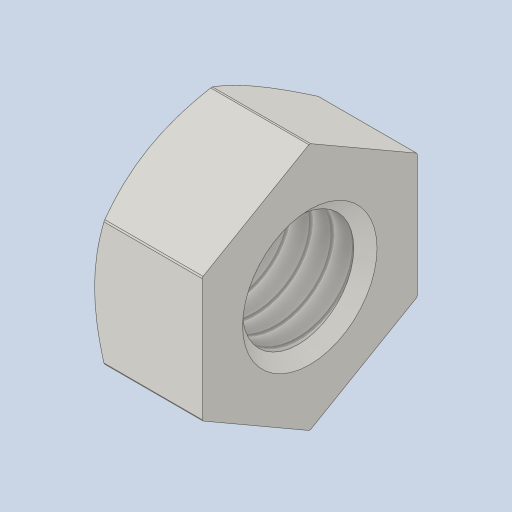
# Autodesk Inventor part: SLBNR5
Saved by Autodesk Inventor 2023 (Build 270158000, 158)
## iProperties
Category: PARTsolutions
Company: MISUMI
Created: 2024-11-13
Part Number: SLBNR5
Material: 鋼
Catalog Web Link: www.cadenas.de
Description: LBNR, LBNL, SLBNR, SLBNL, KNTR, KNTL, SKNTR-Nuts
Vendor: MISUMI
Document SubType Name: Modeling
Designer: psAdmin
Manufacturer: MISUMI
Mass: 1.29398 g
Surface Area: 2.37881 cm^2
Volume: 0.164839 cm^3
Density: 7.85 g/cm^3
Appearance: 鋼
PSOL_IDENT_0: {$CADENAS_DATA/23d-libs/misumi/metric/27_screws_nuts/slbnl.prj},199 {VTYP=3D},{NB=SLBNR5},{LINA=SLBN
PSOL_IDENT_1: R5},{NN=LBNR, LBNL, SLBNR, SLBNL, KNTR, KNTL, SKNTR},{DATE=30.06.2021 13:09:40},{GEOMDATE=05.11.2010
PSOL_IDENT_2: 00:00:00},{VERSION=},{LINEID=40},{WBVAR=TRS,MAT,CS},{WBNUMERIC=}  {NB=SLBNR5},{LINA=SLBNR5},{KT=DUM
PSOL_IDENT_3: MY},{PN=SLBNR5},{TS=LBN},{TRS=R},{MAT=S},{ST=-},{CS=1},{M1=5},{M=5.0},{P=0.80},{B=8.0},{EE=9.2},{T=4
PSOL_IDENT_4: .0},{T1=0.0},{TFX=4.0},{T1FX=3.2},{CALG='1','JIS Class 1','2','JIS Class 3'},{TRSALG= 'R', 'Right-Ha
PSOL_IDENT_5: nd Thread', 'L', 'Left-Hand Thread' },{MATALG= '', 'SWCH Carbon Steel', 'S', '304 Stainless Steel' }
NB: SLBNR5
NN: LBNR, LBNL, SLBNR, SLBNL, KNTR, KNTL, SKNTR
NT: Nuts
NBSYN: $PN.
LINA: SLBNR5
CATALOG: Misumi
PN: SLBNR5
TRS: Right-Hand Thread
MAT: 304 Stainless Steel Equivalent
ST: -
CS: JIS Class 1
M1: 5
P: 0.8
B: 8
EE: 9.2
T: 4
T1: 0
SUPPLIER: MISUMI
ARTICLENO: SLBNR5
BOMINFO: SLBNR5
CREATOR: CADENAS GmbH
Title: SLBNR5
Author: Cadenas PARTsolutions
Comments: Nuts
Autodesk Inventor part; units mm, degrees
sketch "Sketch_1" plane through (0, 0, 0) normal (0, 0, 1) x (1, 0, 0)
  line L0 (2, 0) -> (-2, 0)
  line L1 (-2, 0) -> (-2, 4)
  line L2 (-2, 4) -> (-1.6536, 4.6)
  line L3 (-1.6536, 4.6) -> (2, 4.6)
  line L4 (2, 4.6) -> (2, 0)
  line L5 (2, 0) -> (-2, 0)
  constraints: 12 end point
revolve "Revolution1" add sketch "Sketch_1" angle 360 about axis through (2, 0, 0) along (1, 0, 0)
sketch "Sketch_2" plane through (0, 0, 0) normal (0, 0, 1) x (1, 0, 0)
  line L0 (2, 0) -> (-2, 0)
  line L1 (-2, 0) -> (-2, 2.5)
  line L2 (-2, 2.5) -> (-1.567, 2.067)
  line L3 (-1.567, 2.067) -> (1.567, 2.067)
  line L4 (1.567, 2.067) -> (2, 2.5)
  line L5 (2, 2.5) -> (2, 0)
  line L6 (2, 0) -> (-2, 0)
  constraints: 14 end point
revolve "Revolution2" cut sketch "Sketch_2" angle 360 about axis through (2, 0, 0) along (1, 0, 0)
thread "Thread1" size "M5x0.8" class "6H" standard "ISO Metric profile" full length
sketch "Sketch_3" plane through (0, 0, 0) normal (1, 0, 0) x (0, 1, 0)
  line L0 (-8, 8) -> (-8, -8)
  line L1 (-8, -8) -> (8, -8)
  line L2 (8, -8) -> (8, 8)
  line L3 (8, 8) -> (-8, 8)
  line L4 (-2.3094, 4) -> (-4.6188, 0)
  line L5 (-4.6188, 0) -> (-2.3094, -4)
  line L6 (-2.3094, -4) -> (2.3094, -4)
  line L7 (2.3094, -4) -> (4.6188, 0)
  line L8 (4.6188, 0) -> (2.3094, 4)
  line L9 (2.3094, 4) -> (-2.3094, 4)
  constraints: 20 end point
extrude "Extrusion1" cut sketch "Sketch_3" along normal mid plane 4
ref_plane "cp_XY" through (2, 0, 0) normal (1, 0, 0) x (0, 0, -1)
ref_plane "cp_YZ" through (2, 0, 0) normal (0, 0, -1) x (0, 1, 0)
ref_plane "cp_ZX" through (2, 0, 0) normal (0, 1, 0) x (1, 0, 0)
ref_plane "nut_to_screw_XY" through (0, 0, 0) normal (1, 0, 0) x (0, 0, -1)
ref_plane "nut_to_screw_YZ" through (0, 0, 0) normal (0, 0, -1) x (0, 1, 0)
ref_plane "nut_to_screw_ZX" through (0, 0, 0) normal (0, 1, 0) x (1, 0, 0)
body "Solid1"
